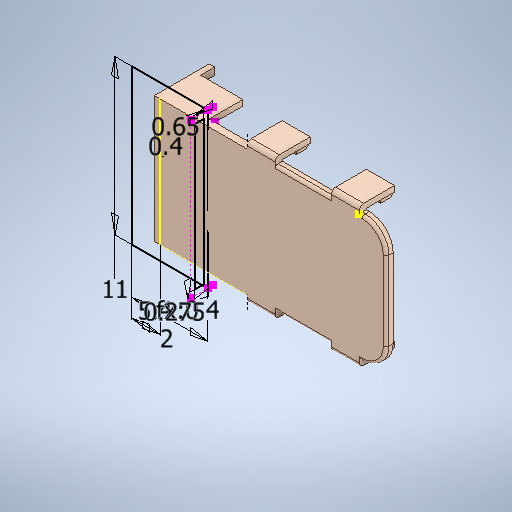
# Autodesk Inventor part: np2alpha_cap_flex_top
Saved by Autodesk Inventor 2025 (Build 290162000, 162)
## iProperties
Created: 2023-07-10
Part Number: np2alpha_cap_flex_top
Material: Generic
Document SubType Name: Modeling
Designer: joao
Density: 1 g/cm^3
Appearance: Default
Author: joao
Autodesk Inventor part; units mm, degrees
ref_plane "Work Plane1" through (-1, 0, 0) normal (0, 0, 1) x (1, 0, 0)
sketch "Sketch1" plane through (-1, 0, 0) normal (0, 0, 1) x (1, 0, 0)
  line L0 (-7, 0) -> (-5, 0)
  line L1 (-5, 0) -> (-5, 0.5)
  line L2 (-5, 0.5) -> (-7, 0.5)
  line L3 (-7, 0.5) -> (-7, 0)
  line L4 (-5, 0) -> (-5, -0.4) projected
  line L5 (-7, 0) -> (-7, -0.4) projected
  line L6 (-1, 0) -> (-1, -0.4) projected
  line L7 (1, 0) -> (1, -0.4) projected
  line L8 (1, -8.6) -> (1, -9) projected
  line L9 (-1, -8.6) -> (-1, -9) projected
  line L10 (-5, -8.6) -> (-5, -9) projected
  line L11 (-7, -8.6) -> (-7, -9) projected
  line L12 (-7, -9.5) -> (-5, -9.5)
  line L13 (-5, -9.5) -> (-5, -9)
  line L14 (-5, -9) -> (-7, -9)
  line L15 (-7, -9) -> (-7, -9.5)
  line L16 (-1, -9.5) -> (1, -9.5)
  line L17 (1, -9.5) -> (1, -9)
  line L18 (1, -9) -> (-1, -9)
  line L19 (-1, -9) -> (-1, -9.5)
  line L20 (-1, 0) -> (1, 0)
  line L21 (1, 0) -> (1, 0.5)
  line L22 (1, 0.5) -> (-1, 0.5)
  line L23 (-1, 0.5) -> (-1, 0)
  line L24 (2.4038, -9) -> (-10, -9) projected
  line L25 (2.4038, 0) -> (-10, 0) projected
  line L26 (-13.2, -9) -> (2.9, -9)
  line L27 (2.9, -9) -> (2.9, 0)
  line L28 (2.9, 0) -> (-13.2, 0)
  line L29 (-13.2, 0) -> (-13.2, -9)
  line L30 (2.7, -2.7) -> (2.7, -1.9958) projected
  line L31 (-13, -9) -> (-13, -5.4522) projected
  point P0 (0.7, -9)
  point P1 (1, 0)
  point P2 (-1, 0)
  point P3 (-5, 0)
  point P4 (-7, 0)
  point P5 (1, 0)
  dimension "d89" = 0.5
  dimension "d90" = 0.2
  dimension "d125" = 0.2
  constraints: 40 end point, 11 collinear, 10 parallel, 5 horizontal, 5 perpendicular, 3 equal length, 3 point on line
  measures "d89" distance of L12.end L13.end
  measures "d90" distance between parallel lines of L29 L31
  measures "d125" distance between parallel lines of L27 L30
extrude "main" add sketch "Sketch1" along normal blind 0.5
sketch "Sketch2" plane through (-1, 0, 0) normal (0, 0, -1) x (-1, 0, 0)
  line L0 (13, 0) -> (-2.4038, 0) projected
  line L1 (-2.4038, -9) -> (13, -9) projected
  line L2 (7, 0.5) -> (7, 0) projected
  line L3 (5, 0) -> (5, 0.5) projected
  line L4 (-1, 0) -> (-1, 0.5) projected
  line L5 (1, 0.5) -> (-1, 0.5)
  line L6 (-1, 0.5) -> (-1, 0.1)
  line L7 (-1, 0.1) -> (1, 0.1)
  line L8 (1, 0.1) -> (1, 0.5)
  line L9 (7, -9) -> (7, -9.5) projected
  line L10 (7, -9.5) -> (5, -9.5)
  line L11 (5, -9.5) -> (5, -9.1)
  line L12 (5, -9.1) -> (7, -9.1)
  line L13 (7, -9.1) -> (7, -9.5)
  line L14 (-1, -9.5) -> (-1, -9) projected
  line L15 (1, -9) -> (1, -9.5) projected
  line L16 (-1, -9.5) -> (1, -9.5)
  line L17 (1, -9.5) -> (1, -9.1)
  line L18 (1, -9.1) -> (-1, -9.1)
  line L19 (-1, -9.1) -> (-1, -9.5)
  line L20 (5, 0.5) -> (7, 0.5) projected
  line L21 (7, 0.5) -> (5, 0.5)
  line L22 (5, 0.5) -> (5, 0.1)
  line L23 (5, 0.1) -> (7, 0.1)
  line L24 (7, 0.1) -> (7, 0.5)
  line L25 (1, 0.5) -> (1, 0) projected
  line L26 (-1, 0.5) -> (1, 0.5) projected
  point P0 (1, -9.5)
  point P1 (-1, -9.1)
  point P2 (-1, 0.5)
  dimension "d91" = 0.1
  dimension "d92" = 0.1
  dimension "d93" = 0.1
  dimension "d94" = 0.1
  constraints: 32 end point, 8 parallel, 4 horizontal, 4 perpendicular, 3 point on line, 2 collinear
  measures "d91" distance between parallel lines of L0 L23
  measures "d92" distance between parallel lines of L0 L7
  measures "d93" distance between parallel lines of L1 L12
  measures "d94" distance between parallel lines of L1 L18
extrude "flaps" add sketch "Sketch2" along normal blind 2 contours L23 L3 L20 L2 | L7 L4 L5 L8 | L9 L10 L11 L12 | L18 L15 L16 L14
sketch "Sketch18" plane through (-1, 0, 0) normal (0, 0, -1) x (-1, 0, 0)
  line L0 (7, 0) -> (13.2, 0) projected
  line L1 (13.2, 0) -> (10.2, 0)
  line L2 (10.2, 0) -> (10.2, -0.4)
  line L3 (10.2, -0.4) -> (13.2, -0.4)
  line L4 (13.2, -0.4) -> (13.2, 0)
  line L5 (13.2, -9) -> (7, -9) projected
  line L6 (13.2, -9) -> (10.2, -9)
  line L7 (10.2, -9) -> (10.2, -8.6)
  line L8 (10.2, -8.6) -> (13.2, -8.6)
  line L9 (13.2, -8.6) -> (13.2, -9)
  line L10 (10, 0) -> (10, -0.4) projected
  line L11 (-1.3, -0.4) -> (10, -0.4) projected
  line L12 (-1.3, -8.6) -> (10, -8.6) projected
  point P0 (-1, 0)
  point P1 (10.2, 0)
  dimension "d95" = 0.2
  constraints: 16 end point, 4 parallel, 2 collinear, 2 horizontal, 2 perpendicular, 1 point on line
  measures "d95" distance between parallel lines of L10 L2
extrude "Extrusion18" add sketch "Sketch18" along normal blind 2.4
ref_plane "Work Plane4" through (-14.2, -9, 0.5) normal (-1, 0, 0) x (0, 0, 1)
sketch "Sketch19" plane through (-14.2, -9, 0.5) normal (-1, 0, 0) x (0, 0, 1)
  line L0 (0, 9) -> (0, 0) projected
  line L1 (0, 9) -> (-3.9, 9)
  line L2 (-3.9, 9) -> (-3.9, 0)
  line L3 (-3.9, 0) -> (0, 0)
  line L4 (0, 0) -> (0, 9)
  line L5 (-3.9, 8.5) -> (-3.9, 0.5) projected
  constraints: 8 end point, 2 parallel, 1 collinear, 1 horizontal, 1 perpendicular
extrude "Extrusion19" add sketch "Sketch19" along normal blind 0.4
fillet "Fillet7" radius 0.3 4 edges at (-1, -9.5, 0.5) (-1, 0.5, 0.5) (-7, 0.5, 0.5) (-7, -9.5, 0.5)
fillet "Fillet9" radius 1.7 2 edges at (1.9, 0, 0.25) (1.9, -9, 0.25)
sketch "Sketch22" plane through (-8, -9.1, 0) normal (0, 1, 0) x (1, 0, 0)
  line L0 (0, 0.9) -> (2, 0.9) projected
  line L1 (0, 2.1) -> (0, 0.9) projected
  line L2 (2, 0.9) -> (2, 2.1) projected
  line L3 (6, 0.9) -> (8, 0.9) projected
  line L4 (8, 0.9) -> (8, 2.1) projected
  line L5 (6, 2.1) -> (8, 2.1) projected
  line L6 (6, 2.1) -> (6, 0.9) projected
  line L7 (2, 2.1) -> (0, 2.1) projected
  line L8 (0.1, 1.1) -> (1.9, 1.1)
  line L9 (1.9, 1.1) -> (1.9, 2)
  line L10 (1.9, 2) -> (0.1, 2)
  line L11 (0.1, 2) -> (0.1, 1.1)
  line L12 (6.1, 1.1) -> (7.9, 1.1)
  line L13 (7.9, 1.1) -> (7.9, 2)
  line L14 (7.9, 2) -> (6.1, 2)
  line L15 (6.1, 2) -> (6.1, 1.1)
  point P0 (8, 0)
  dimension "d134" = 0.1
  dimension "d135" = 0.2
  dimension "d136" = 0.1
  dimension "d137" = 0.1
  dimension "d138" = 0.1
  dimension "d139" = 0.1
  dimension "d140" = 0.1
  constraints: 16 end point, 4 parallel, 2 horizontal, 2 perpendicular, 1 point on line
  measures "d134" distance between parallel lines of L7 L10
  measures "d135" distance between parallel lines of L0 L8
  measures "d136" distance between parallel lines of L2 L9
  measures "d137" distance between parallel lines of L1 L11
  measures "d138" distance between parallel lines of L5 L14
  measures "d139" distance between parallel lines of L6 L15
  measures "d140" distance between parallel lines of L4 L13
extrude "Extrusion22" add sketch "Sketch22" along normal blind 0.3 contours L11 L10 L9 L8 | L15 L14 L13 L12
sketch "Sketch23" plane through (-2, 0.1, 0) normal (0, -1, 0) x (1, 0, 0)
  line L0 (1.9, -2) -> (0.1, -2) projected
  line L1 (0.1, -1.1) -> (1.9, -1.1) projected
  line L2 (0.1, -2) -> (0.1, -1.1) projected
  line L3 (1.9, -1.1) -> (1.9, -2) projected
  line L4 (-4.1, -1.1) -> (-4.1, -2) projected
  line L5 (-4.1, -2) -> (-5.9, -2) projected
  line L6 (-5.9, -1.1) -> (-4.1, -1.1) projected
  line L7 (-5.9, -2) -> (-5.9, -1.1) projected
  point P0 (2, 0)
extrude "Extrusion23" add sketch "Sketch23" along normal blind 0.3
chamfer "Chamfer6" distance 0.2 angle 45 4 edges at (-1, -8.8, -2) (-7, -8.8, -2) (-7, -0.2, -2) (-1, -0.2, -2)
fillet "Fillet11" radius 0.2 5 edges at (1.4021, -0.4979, 0.5) (1.4021, -8.5021, 0.5) (1.9, -4.5, 0.5) (-4, -9, 0.5) (-4, 0, 0.5)
sketch "Sketch9" plane through (-1, 0, 0.5) normal (0, 0, 1) x (1, 0, 0)
  line L0 (-15.2, -10) -> (-9.8, -10)
  line L1 (-9.8, -10) -> (-9.8, 1)
  line L2 (-9.8, 1) -> (-15.2, 1)
  line L3 (-15.2, 1) -> (-15.2, -10)
  line L4 (-13.2, 0) -> (-13.2, -9) projected
  line L5 (-13.2, -9) -> (-7, -9) construction
  line L6 (-7, -9) -> (-7, -10) construction
  line L7 (-7, 0.1) -> (-7, 0) construction
  line L8 (-7, 0) -> (-7, 1) construction
  point P0 (1, 0)
  dimension "d100" = 5.4
  dimension "d101" = 11
  dimension "d102" = 2
  constraints: 12 end point, 3 perpendicular, 2 parallel, 2 point on line, 1 collinear, 1 horizontal
  measures "d100" distance of L0.start L0.end
  measures "d101" distance of L2.end L0.start
  measures "d102" distance between parallel lines of L3 L4
ref_plane "Work Plane3" through (-10.8, -9.5, 0.5) normal (1, 0, 0) x (0, 0, -1)
sketch "Sketch20" plane through (-10.8, -9.5, 0.5) normal (1, 0, 0) x (0, 0, -1)
  line L0 (-0.925, -0.1) -> (-0.275, -0.1)
  line L1 (-0.275, -0.1) -> (-0.275, 10.1)
  line L2 (-0.275, 10.1) -> (-0.925, 10.1)
  line L3 (-0.925, 10.1) -> (-0.925, -0.1)
  line L4 (0, -0.5) -> (-1.2, -0.5) construction
  line L5 (0, 10.5) -> (-1.2, 10.5) construction
  line L6 (-1.2, -0.5) -> (-1.2, 10.5) construction
  point P0 (0.5, 9.5)
  point P1 (0.4, -0.5)
  point P2 (0.4, 10.5)
  dimension "d105" = 0.275
  dimension "d106" = 0.65
  dimension "d107" = 0.4
  dimension "d108" = 0.4
  constraints: 8 end point, 2 parallel, 1 horizontal, 1 perpendicular
  measures "d105" distance between parallel lines of L6 L3
  measures "d106" distance between parallel lines of L3 L1
  measures "d107" distance between parallel lines of L5 L2
  measures "d108" distance between parallel lines of L4 L0
sketch "Sketch24" plane through (-14.6, -9, 0.5) normal (-1, 0, 0) x (0, 0, 1)
  line L0 (-4.7023, 8.5) -> (-3.4, 8.5)
  line L1 (-3.4, 8.5) -> (-3.4, 0.5)
  line L2 (-3.4, 0.5) -> (-4.7023, 0.5)
  line L3 (-4.7023, 0.5) -> (-4.7023, 8.5)
  line L4 (0, 0) -> (0, 9) projected
  line L5 (0, 9) -> (-3.9, 9) projected
  line L6 (-3.9, 9) -> (-3.9, 0) projected
  line L7 (-3.9, 0) -> (0, 0) projected
  point P0 (-0.5, 9)
  point P1 (-4.0512, 8.5)
  dimension "d152" = 8
  dimension "d153" = 0.5
  dimension "d154" = 0.5
  constraints: 8 end point, 2 parallel, 1 horizontal, 1 midpoint, 1 perpendicular
  measures "d152" distance between parallel lines of L2 L0
  measures "d153" distance from line of L5 point (-4.051, 8.5)
  measures "d154" distance between parallel lines of L1 L6
extrude "Extrusion24" cut sketch "Sketch24" against normal blind 10 contours L0 L6 L2 L3 | L0 L1 L2 L6
body "Solid1"
